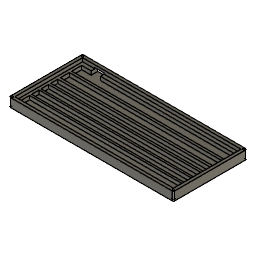
_Bottom_Mech_Case.80a9186b-1b8e-4eee-9d71-97a39b245fca (Autodesk Fusion 360 design; units mm, degrees)
part number: 2026-01-07-15-56-08-248
part number: 2026-01-07-15-57-18-845
Autodesk Fusion 360 part; units mm, degrees
(part 1 of 2)
sketch "Sketch1" plane through (0, 0, 0) normal (0, 0, 1) x (1, 0, 0) in component "MechKeyboard"
  line L0 (0, 0) -> (317.706, 0)
  line L1 (317.706, 0) -> (317.706, 135.488)
  line L2 (317.706, 135.488) -> (0, 135.488)
  line L3 (0, 135.488) -> (0, 0)
  line L4 (-6, -6) -> (323.706, -6)
  line L5 (323.706, -6) -> (323.706, 141.488)
  line L6 (323.706, 141.488) -> (-6, 141.488)
  line L7 (-6, 141.488) -> (-6, -6)
  circle A0 centre (320.206, 137.988) radius 1.7
  circle A1 centre (320.206, 137.988) radius 3
  line L8 (158.853, 135.488) -> (158.853, 141.488) construction
  line L9 (317.706, 67.744) -> (323.706, 67.744) construction
  circle A2 centre (320.206, -2.5) radius 3
  circle A3 centre (320.206, -2.5) radius 1.7
  circle A4 centre (-2.5, 137.988) radius 1.7
  circle A5 centre (-2.5, 137.988) radius 3
  circle A6 centre (-2.5, -2.5) radius 1.7
  circle A7 centre (-2.5, -2.5) radius 3
  dimension "d1" = 317.706
  dimension "d2" = 135.488
  dimension "d3" = 6
  dimension "d4" = 3.4
  dimension "d5" = 3.5
  dimension "d6" = 3.5
  dimension "d7" = 6
  constraint horizontal L0
  constraint vertical L1
  constraint horizontal L2
  constraint vertical L3
  constraint coincident L0.start L3.end
  constraint concentric A0 A1
  constraint midpoint L2 L8.start
  constraint midpoint L6 L8.end
  constraint midpoint L1 L9.start
  constraint midpoint L5 L9.end
  constraint symmetric A0 L9 A3
  constraint symmetric A1 L9 A2
  constraint symmetric A0 L8 A4
  constraint symmetric A1 L8 A5
  constraint symmetric L8 A2 A7
  constraint symmetric L8 A3 A6
  measures "d1" distance of L0.start L0.end
  measures "d2" distance of L0.end L1.end
  measures "d4" diameter of A0
  measures "d5" distance of L5 A0.centre
  measures "d6" distance of L6 A0.centre
  measures "d7" diameter of A1
extrude "Extrude1" add sketch "Sketch1" along normal blind 14.4 from surface at 3.1 contours A1 | A2 | A5 | A7 makes body 1 at (0.4851, -2.7987, 7.9) makes body 2 at (318.8374, 0.1696, 12.7) makes body 3 at (-5.3191, 139.0141, 12.7) makes body 4 at (321.4399, 140.7225, 12.7) in component "MechKeyboard"
extrude "Extrude2" add sketch "Sketch1" along normal blind 17.5 contours L4 L5 L6 L7 bodies 1 2 3 4 in component "MechKeyboard"
extrude "Extrude3" add sketch "Sketch1" along normal blind 3 contours L0 L1 L2 L3 bodies 1 in component "MechKeyboard"
sketch "Sketch1 (2)" plane through (0, 0, 17.5) normal (0, 0, 1) x (-1, 0, 0)
  line L0 (0, 0) -> (0, -135.488)
  line L1 (0, -135.488) -> (-317.706, -135.488)
  line L2 (-317.706, -135.488) -> (-317.706, 0)
  line L3 (-317.706, 0) -> (0, 0)
  line L4 (6, -141.488) -> (6, 6)
  line L5 (6, 6) -> (-323.706, 6)
  line L6 (-323.706, 6) -> (-323.706, -141.488)
  line L7 (-323.706, -141.488) -> (6, -141.488)
  line L8 (-24.5, -141.488) -> (-43, -141.488)
  line L9 (-43, -141.488) -> (-43, -135.488)
  line L10 (-43, -135.488) -> (-24.5, -135.488)
  line L11 (-24.5, -135.488) -> (-24.5, -141.488)
  circle A0 centre (2.5, 2.5) radius 1.7
  circle A1 centre (-320.206, -137.988) radius 1.7
  circle A2 centre (-320.206, 2.5) radius 1.7
  circle A3 centre (2.5, -137.988) radius 1.7
  dimension "d15" = 18.5
  dimension "d17" = 24.5
  constraint horizontal L8
  constraint vertical L9
  constraint horizontal L10
  constraint vertical L11
  constraint coincident L1 L9.end
  constraint coincident L7 L8.start
  measures "d15" distance of L9 L11
  measures "d17" distance of L0.end L11
extrude "Extrude4" cut sketch "Sketch1 (2)" against normal up to surface (9.5 mm away) from surface at -5 contours L1 L7 L8 L9 L10 L11 bodies 1 in component "MechKeyboard"
fillet "Fillet1" radius 2.5 4 edges at (-6, 141.488, 8.75) (-6, -6, 8.75) (323.706, -6, 8.75) (323.706, 141.488, 8.75) on bodies 1 in component "MechKeyboard"
sketch "Sketch2" plane through (0, 0, 3) normal (0, 0, 1) x (-1, 0, 0)
  line L0 (-95.203, -110.7503, 10) -> (-108.203, -110.7503, 10)
  arc A0 through (-232.028, -10.7378, 10) (-232.3816, -10.8842, 10) (-232.528, -11.2378, 10)
  arc A1 through (-184.4218, -23.7378, 10) (-184.0682, -23.5913, 10) (-183.9218, -23.2378, 10)
  arc A2 through (-270.128, -10.7378, 10) (-270.4816, -10.8842, 10) (-270.628, -11.2378, 10)
  arc A3 through (-58.9843, -11.2378, 10) (-59.1307, -10.8842, 10) (-59.4843, -10.7378, 10)
  arc A4 through (-183.9218, -9.2378, 10) (-184.0682, -8.8842, 10) (-184.4218, -8.7378, 10)
  arc A5 through (-308.228, -10.7378, 10) (-308.5816, -10.8842, 10) (-308.728, -11.2378, 10)
  arc A6 through (-251.078, -10.7378, 10) (-251.4316, -10.8842, 10) (-251.578, -11.2378, 10)
  arc A7 through (-11.3593, -11.2378, 10) (-11.5057, -10.8842, 10) (-11.8593, -10.7378, 10)
  arc A8 through (-308.728, -24.2378, 10) (-308.5816, -24.5913, 10) (-308.228, -24.7378, 10)
  arc A9 through (-190.4218, -8.7378, 10) (-190.7753, -8.8842, 10) (-190.9218, -9.2378, 10)
  arc A10 through (-256.628, -11.2378, 10) (-256.7744, -10.8842, 10) (-257.128, -10.7378, 10)
  arc A11 through (-130.4218, -11.2378, 10) (-130.5682, -10.8842, 10) (-130.9218, -10.7378, 10)
  circle A12 through (-323.206, 2.5, 10) (-318.706, -0.0981, 10) (-318.706, 5.0981, 10)
  arc A13 through (-25.3593, -24.2378, 10) (-25.2128, -24.5913, 10) (-24.8593, -24.7378, 10)
  arc A14 through (-275.678, -30.2878, 10) (-275.8244, -29.9342, 10) (-276.178, -29.7878, 10)
  arc A15 through (-289.178, -29.7878, 10) (-289.5316, -29.9342, 10) (-289.678, -30.2878, 10)
  arc A16 through (-295.228, -24.7378, 10) (-294.8744, -24.5913, 10) (-294.728, -24.2378, 10)
  arc A17 through (-294.728, -11.2378, 10) (-294.8744, -10.8842, 10) (-295.228, -10.7378, 10)
  arc A18 through (-295.228, -43.7878, 10) (-294.8744, -43.6413, 10) (-294.728, -43.2878, 10)
  arc A19 through (-289.678, -43.2878, 10) (-289.5316, -43.6413, 10) (-289.178, -43.7878, 10)
  arc A20 through (-185.6905, -43.7878, 10) (-185.3369, -43.6413, 10) (-185.1905, -43.2878, 10)
  arc A21 through (-18.9463, -27.7878, 10) (-19.2998, -27.9342, 10) (-19.4463, -28.2878, 10)
  arc A22 through (-276.178, -43.7878, 10) (-275.8244, -43.6413, 10) (-275.678, -43.2878, 10)
  arc A23 through (-12.9463, -42.7878, 10) (-12.5927, -42.6413, 10) (-12.4463, -42.2878, 10)
  arc A24 through (-249.9843, -43.7878, 10) (-249.6307, -43.6413, 10) (-249.4843, -43.2878, 10)
  arc A25 through (-249.4843, -30.2878, 10) (-249.6307, -29.9342, 10) (-249.9843, -29.7878, 10)
  arc A26 through (-84.3905, -29.7878, 10) (-84.7441, -29.9342, 10) (-84.8905, -30.2878, 10)
  arc A27 through (-83.9218, -9.2378, 10) (-84.0682, -8.8842, 10) (-84.4218, -8.7378, 10)
  arc A28 through (-190.9218, -23.2378, 10) (-190.7753, -23.5913, 10) (-190.4218, -23.7378, 10)
  arc A29 through (-204.2405, -30.2878, 10) (-204.3869, -29.9342, 10) (-204.7405, -29.7878, 10)
  arc A30 through (-143.9218, -10.7378, 10) (-144.2753, -10.8842, 10) (-144.4218, -11.2378, 10)
  arc A31 through (-185.1905, -30.2878, 10) (-185.3369, -29.9342, 10) (-185.6905, -29.7878, 10)
  arc A32 through (-103.9405, -43.2878, 10) (-103.7941, -43.6413, 10) (-103.4405, -43.7878, 10)
  arc A33 through (-48.6718, -10.7378, 10) (-49.0253, -10.8842, 10) (-49.1718, -11.2378, 10)
  arc A34 through (-170.6155, -62.3378, 10) (-170.4691, -62.6913, 10) (-170.1155, -62.8378, 10)
  arc A35 through (-65.3405, -29.7878, 10) (-65.6941, -29.9342, 10) (-65.8405, -30.2878, 10)
  arc A36 through (-279.7098, -61.8378, 10) (-279.3562, -61.6913, 10) (-279.2098, -61.3378, 10)
  arc A37 through (-232.8155, -49.3378, 10) (-232.9619, -48.9842, 10) (-233.3155, -48.8378, 10)
  arc A38 through (-308.728, -62.3378, 10) (-308.5816, -62.6913, 10) (-308.228, -62.8378, 10)
  arc A39 through (-217.7405, -29.7878, 10) (-218.0941, -29.9342, 10) (-218.2405, -30.2878, 10)
  arc A40 through (-118.5155, -49.3378, 10) (-118.6619, -48.9842, 10) (-119.0155, -48.8378, 10)
  arc A41 through (-219.028, -24.7378, 10) (-218.6744, -24.5913, 10) (-218.528, -24.2378, 10)
  arc A42 through (-208.7155, -62.3378, 10) (-208.5691, -62.6913, 10) (-208.2155, -62.8378, 10)
  arc A43 through (-113.4655, -62.3378, 10) (-113.3191, -62.6913, 10) (-112.9655, -62.8378, 10)
  arc A44 through (-198.6905, -29.7878, 10) (-199.0441, -29.9342, 10) (-199.1905, -30.2878, 10)
  arc A45 through (-29.6218, -48.8378, 10) (-29.9753, -48.9842, 10) (-30.1218, -49.3378, 10)
  arc A46 through (-212.978, -10.7378, 10) (-213.3316, -10.8842, 10) (-213.478, -11.2378, 10)
  arc A47 through (-180.1405, -43.2878, 10) (-179.9941, -43.6413, 10) (-179.6405, -43.7878, 10)
  arc A48 through (-80.4155, -49.3378, 10) (-80.5619, -48.9842, 10) (-80.9155, -48.8378, 10)
  arc A49 through (-61.8655, -62.8378, 10) (-61.5119, -62.6913, 10) (-61.3655, -62.3378, 10)
  arc A50 through (-99.9655, -62.8378, 10) (-99.6119, -62.6913, 10) (-99.4655, -62.3378, 10)
  arc A51 through (-208.2155, -48.8378, 10) (-208.5691, -48.9842, 10) (-208.7155, -49.3378, 10)
  arc A52 through (-209.003, -68.3878, 10) (-209.1494, -68.0342, 10) (-209.503, -67.8878, 10)
  arc A53 through (-175.6655, -49.3378, 10) (-175.8119, -48.9842, 10) (-176.1655, -48.8378, 10)
  arc A54 through (-90.4218, -8.7378, 10) (-90.7753, -8.8842, 10) (-90.9218, -9.2378, 10)
  arc A55 through (-199.1905, -43.2878, 10) (-199.0441, -43.6413, 10) (-198.6905, -43.7878, 10)
  arc A56 through (-147.0905, -30.2878, 10) (-147.2369, -29.9342, 10) (-147.5905, -29.7878, 10)
  arc A57 through (-228.053, -68.3878, 10) (-228.1994, -68.0342, 10) (-228.553, -67.8878, 10)
  arc A58 through (-16.6218, -62.8378, 10) (-16.2682, -62.6913, 10) (-16.1218, -62.3378, 10)
  arc A59 through (-72.4843, -10.7378, 10) (-72.8378, -10.8842, 10) (-72.9843, -11.2378, 10)
  arc A60 through (-270.9155, -68.3878, 10) (-271.0619, -68.0342, 10) (-271.4155, -67.8878, 10)
  arc A61 through (-246.3155, -48.8378, 10) (-246.6691, -48.9842, 10) (-246.8155, -49.3378, 10)
  arc A62 through (-223.7905, -43.7878, 10) (-223.4369, -43.6413, 10) (-223.2905, -43.2878, 10)
  arc A63 through (-228.553, -81.8878, 10) (-228.1994, -81.7413, 10) (-228.053, -81.3878, 10)
  arc A64 through (-190.453, -81.8878, 10) (-190.0994, -81.7413, 10) (-189.953, -81.3878, 10)
  arc A65 through (-95.203, -81.8878, 10) (-94.8494, -81.7413, 10) (-94.703, -81.3878, 10)
  arc A66 through (-166.6405, -43.7878, 10) (-166.2869, -43.6413, 10) (-166.1405, -43.2878, 10)
  arc A67 through (-165.353, -67.8878, 10) (-165.7066, -68.0342, 10) (-165.853, -68.3878, 10)
  arc A68 through (-170.1155, -48.8378, 10) (-170.4691, -48.9842, 10) (-170.6155, -49.3378, 10)
  arc A69 through (-90.4405, -43.7878, 10) (-90.0869, -43.6413, 10) (-89.9405, -43.2878, 10)
  arc A70 through (-89.153, -67.8878, 10) (-89.5066, -68.0342, 10) (-89.653, -68.3878, 10)
  arc A71 through (-146.303, -67.8878, 10) (-146.6566, -68.0342, 10) (-146.803, -68.3878, 10)
  arc A72 through (-38.053, -81.8878, 10) (-37.6994, -81.7413, 10) (-37.553, -81.3878, 10)
  arc A73 through (-70.103, -67.8878, 10) (-70.4566, -68.0342, 10) (-70.603, -68.3878, 10)
  arc A74 through (-146.803, -81.3878, 10) (-146.6566, -81.7413, 10) (-146.303, -81.8878, 10)
  arc A75 through (-132.0155, -48.8378, 10) (-132.3691, -48.9842, 10) (-132.5155, -49.3378, 10)
  line L1 (-58.9843, -24.2378, 10) -> (-58.9843, -11.2378, 10)
  line L2 (-72.9843, -24.2378, 10) -> (-72.9843, -11.2378, 10)
  arc A76 through (-70.603, -81.3878, 10) (-70.4566, -81.7413, 10) (-70.103, -81.8878, 10)
  arc A77 through (-95.203, -124.7503, 10) (-94.8494, -124.6038, 10) (-94.703, -124.2503, 10)
  arc A78 through (-89.653, -124.2503, 10) (-89.5066, -124.6038, 10) (-89.153, -124.7503, 10)
  line L3 (-190.9218, -23.2378, 10) -> (-190.9218, -9.2378, 10)
  arc A79 through (-165.853, -81.3878, 10) (-165.7066, -81.7413, 10) (-165.353, -81.8878, 10)
  line L4 (-59.4843, -24.7378, 10) -> (-72.4843, -24.7378, 10)
  arc A80 through (-209.503, -81.8878, 10) (-209.1494, -81.7413, 10) (-209.003, -81.3878, 10)
  arc A81 through (-57.103, -124.7503, 10) (-56.7494, -124.6038, 10) (-56.603, -124.2503, 10)
  arc A82 through (-127.753, -81.3878, 10) (-127.6066, -81.7413, 10) (-127.253, -81.8878, 10)
  line L5 (-84.4218, -8.7378, 10) -> (-90.4218, -8.7378, 10)
  line L6 (-35.6718, -24.7378, 10) -> (-48.6718, -24.7378, 10)
  line L7 (-256.628, -24.2378, 10) -> (-256.628, -11.2378, 10)
  arc A83 through (-264.215, -84.9378, 10) (-264.5686, -85.0842, 10) (-264.715, -85.4378, 10)
  line L8 (-323.706, 6, 10) -> (-323.706, -141.488, 10)
  arc A84 through (-232.528, -100.4378, 10) (-232.3816, -100.7913, 10) (-232.028, -100.9378, 10)
  arc A85 through (-266.153, -87.4378, 10) (-266.2994, -87.0842, 10) (-266.653, -86.9378, 10)
  line L9 (-289.678, -43.2878, 10) -> (-289.678, -30.2878, 10)
  line L10 (-275.678, -43.2878, 10) -> (-275.678, -30.2878, 10)
  line L11 (-289.678, -24.2378, 10) -> (-289.678, -11.2378, 10)
  line L12 (-90.9218, -23.2378, 10) -> (-90.9218, -9.2378, 10)
  line L13 (-59.4843, -10.7378, 10) -> (-72.4843, -10.7378, 10)
  arc A86 through (-123.278, -87.4378, 10) (-123.4244, -87.0842, 10) (-123.778, -86.9378, 10)
  line L14 (-183.9218, -23.2378, 10) -> (-183.9218, -9.2378, 10)
  line L15 (-223.2905, -43.2878, 10) -> (-223.2905, -30.2878, 10)
  line L16 (-180.1405, -43.2878, 10) -> (-180.1405, -30.2878, 10)
  line L17 (-204.2405, -43.2878, 10) -> (-204.2405, -30.2878, 10)
  line L18 (-218.2405, -43.2878, 10) -> (-218.2405, -30.2878, 10)
  line L19 (-308.728, -43.2878, 10) -> (-308.728, -30.2878, 10)
  arc A87 through (-161.378, -87.4378, 10) (-161.5244, -87.0842, 10) (-161.878, -86.9378, 10)
  arc A88 through (-47.078, -87.4378, 10) (-47.2244, -87.0842, 10) (-47.578, -86.9378, 10)
  line L20 (-130.4218, -24.2378, 10) -> (-130.4218, -11.2378, 10)
  line L21 (-84.8905, -43.2878, 10) -> (-84.8905, -30.2878, 10)
  line L22 (-36.8223, -42.7878, 10) -> (-42.8223, -42.7878, 10)
  arc A89 through (-8.978, -87.4378, 10) (-9.1244, -87.0842, 10) (-9.478, -86.9378, 10)
  arc A90 through (-22.978, -100.4378, 10) (-22.8316, -100.7913, 10) (-22.478, -100.9378, 10)
  line L23 (-161.0905, -43.2878, 10) -> (-161.0905, -30.2878, 10)
  line L24 (-109.4905, -29.7878, 10) -> (-122.4905, -29.7878, 10)
  line L25 (-128.0405, -43.2878, 10) -> (-128.0405, -30.2878, 10)
  line L26 (-147.5905, -29.7878, 10) -> (-160.5905, -29.7878, 10)
  line L27 (-42.8155, -62.8378, 10) -> (-55.8155, -62.8378, 10)
  line L28 (-70.603, -81.3878, 10) -> (-70.603, -68.3878, 10)
  line L29 (-38.053, -81.8878, 10) -> (-51.053, -81.8878, 10)
  line L30 (-16.1218, -62.3378, 10) -> (-16.1218, -49.3378, 10)
  line L31 (-119.0155, -48.8378, 10) -> (-132.0155, -48.8378, 10)
  line L32 (-11.3593, -24.2378, 10) -> (-11.3593, -11.2378, 10)
  line L33 (-308.728, -81.3878, 10) -> (-308.728, -68.3878, 10)
  line L34 (-157.1155, -48.8378, 10) -> (-170.1155, -48.8378, 10)
  line L35 (-42.3155, -62.3378, 10) -> (-42.3155, -49.3378, 10)
  line L36 (-51.553, -81.3878, 10) -> (-51.553, -68.3878, 10)
  line L37 (-249.9843, -43.7878, 10) -> (-262.9843, -43.7878, 10)
  line L38 (-80.9155, -62.8378, 10) -> (-93.9155, -62.8378, 10)
  line L39 (-109.4905, -43.7878, 10) -> (-122.4905, -43.7878, 10)
  line L40 (-288.591, -99.4378, 10) -> (-288.591, -85.4378, 10)
  line L41 (-30.1218, -62.3378, 10) -> (-30.1218, -49.3378, 10)
  line L42 (-133.303, -81.8878, 10) -> (-146.303, -81.8878, 10)
  line L43 (-266.653, -100.9378, 10) -> (-279.653, -100.9378, 10)
  line L44 (-228.053, -81.3878, 10) -> (-228.053, -68.3878, 10)
  line L45 (-165.853, -81.3878, 10) -> (-165.853, -68.3878, 10)
  line L46 (-12.9463, -42.7878, 10) -> (-18.9463, -42.7878, 10)
  line L47 (-52.3405, -29.7878, 10) -> (-65.3405, -29.7878, 10)
  line L48 (-270.9155, -81.3878, 10) -> (-270.9155, -68.3878, 10)
  line L49 (-76.153, -67.8878, 10) -> (-89.153, -67.8878, 10)
  line L50 (-295.228, -81.8878, 10) -> (-308.228, -81.8878, 10)
  line L51 (-118.228, -100.4378, 10) -> (-118.228, -87.4378, 10)
  line L52 (-295.228, -67.8878, 10) -> (-308.228, -67.8878, 10)
  line L53 (-199.978, -100.9378, 10) -> (-212.978, -100.9378, 10)
  line L54 (-295.228, -86.9378, 10) -> (-308.228, -86.9378, 10)
  line L55 (-99.178, -100.4378, 10) -> (-99.178, -87.4378, 10)
  line L56 (-108.703, -81.3878, 10) -> (-108.703, -68.3878, 10)
  line L57 (-20.8843, -43.2878, 10) -> (-20.8843, -30.2878, 10)
  line L58 (-199.478, -100.4378, 10) -> (-199.478, -87.4378, 10)
  arc A91 through (-289.678, -24.2378, 10) (-289.5316, -24.5913, 10) (-289.178, -24.7378, 10)
  circle A92 through (-0.5, -137.988, 10) (4, -140.5861, 10) (4, -135.3899, 10)
  arc A93 through (-251.078, -86.9378, 10) (-251.4316, -87.0842, 10) (-251.578, -87.4378, 10)
  line L59 (-108.703, -124.2503, 10) -> (-108.703, -111.2503, 10)
  arc A94 through (-281.591, -85.4378, 10) (-281.7374, -85.0842, 10) (-282.091, -84.9378, 10)
  arc A95 through (-257.715, -85.4378, 10) (-257.8614, -85.0842, 10) (-258.215, -84.9378, 10)
  arc A96 through (-42.8155, -62.8378, 10) (-42.4619, -62.6913, 10) (-42.3155, -62.3378, 10)
  arc A97 through (-70.8905, -30.2878, 10) (-71.0369, -29.9342, 10) (-71.3905, -29.7878, 10)
  arc A98 through (-114.253, -81.8878, 10) (-113.8994, -81.7413, 10) (-113.753, -81.3878, 10)
  arc A99 through (-19.4463, -42.2878, 10) (-19.2998, -42.6413, 10) (-18.9463, -42.7878, 10)
  arc A100 through (-65.8405, -43.2878, 10) (-65.6941, -43.6413, 10) (-65.3405, -43.7878, 10)
  arc A101 through (-13.7405, -68.3878, 10) (-13.8869, -68.0342, 10) (-14.2405, -67.8878, 10)
  arc A102 through (-308.228, -67.8878, 10) (-308.5816, -68.0342, 10) (-308.728, -68.3878, 10)
  arc A103 through (-219.028, -100.9378, 10) (-218.6744, -100.7913, 10) (-218.528, -100.4378, 10)
  arc A104 through (-27.7405, -81.3878, 10) (-27.5941, -81.7413, 10) (-27.2405, -81.8878, 10)
  arc A105 through (-295.228, -81.8878, 10) (-294.8744, -81.7413, 10) (-294.728, -81.3878, 10)
  arc A106 through (-34.8843, -43.2878, 10) (-34.7378, -43.6413, 10) (-34.3843, -43.7878, 10)
  arc A107 through (-142.828, -100.9378, 10) (-142.4744, -100.7913, 10) (-142.328, -100.4378, 10)
  arc A108 through (-56.603, -68.3878, 10) (-56.7494, -68.0342, 10) (-57.103, -67.8878, 10)
  arc A109 through (-117.728, -86.9378, 10) (-118.0816, -87.0842, 10) (-118.228, -87.4378, 10)
  arc A110 through (-9.478, -100.9378, 10) (-9.1244, -100.7913, 10) (-8.978, -100.4378, 10)
  arc A111 through (-257.128, -124.7503, 10) (-256.7744, -124.6038, 10) (-256.628, -124.2503, 10)
  arc A112 through (-238.078, -100.9378, 10) (-237.7244, -100.7913, 10) (-237.578, -100.4378, 10)
  arc A113 through (-282.091, -99.9378, 10) (-281.7374, -99.7913, 10) (-281.591, -99.4378, 10)
  line L60 (-9.478, -110.7503, 10) -> (-22.478, -110.7503, 10)
  arc A114 through (-251.578, -100.4378, 10) (-251.4316, -100.7913, 10) (-251.078, -100.9378, 10)
  arc A115 through (-79.628, -86.9378, 10) (-79.9816, -87.0842, 10) (-80.128, -87.4378, 10)
  arc A116 through (-246.8155, -62.3378, 10) (-246.6691, -62.6913, 10) (-246.3155, -62.8378, 10)
  arc A117 through (-157.1155, -62.8378, 10) (-156.7619, -62.6913, 10) (-156.6155, -62.3378, 10)
  arc A118 through (-80.9155, -62.8378, 10) (-80.5619, -62.6913, 10) (-80.4155, -62.3378, 10)
  arc A119 through (-285.7098, -46.8378, 10) (-286.0633, -46.9842, 10) (-286.2098, -47.3378, 10)
  arc A120 through (-261.103, -81.3878, 10) (-260.9566, -81.7413, 10) (-260.603, -81.8878, 10)
  arc A121 through (-264.715, -99.4378, 10) (-264.5686, -99.7913, 10) (-264.215, -99.9378, 10)
  arc A122 through (-41.528, -86.9378, 10) (-41.8816, -87.0842, 10) (-42.028, -87.4378, 10)
  arc A123 through (-258.215, -99.9378, 10) (-257.8614, -99.7913, 10) (-257.715, -99.4378, 10)
  arc A124 through (-42.028, -100.4378, 10) (-41.8816, -100.7913, 10) (-41.528, -100.9378, 10)
  arc A125 through (-176.1655, -62.8378, 10) (-175.8119, -62.6913, 10) (-175.6655, -62.3378, 10)
  arc A126 through (-22.478, -86.9378, 10) (-22.8316, -87.0842, 10) (-22.978, -87.4378, 10)
  arc A127 through (-89.653, -81.3878, 10) (-89.5066, -81.7413, 10) (-89.153, -81.8878, 10)
  arc A128 through (-193.928, -86.9378, 10) (-194.2816, -87.0842, 10) (-194.428, -87.4378, 10)
  arc A129 through (-70.603, -124.2503, 10) (-70.4566, -124.6038, 10) (-70.103, -124.7503, 10)
  arc A130 through (-251.578, -124.2503, 10) (-251.4316, -124.6038, 10) (-251.078, -124.7503, 10)
  arc A131 through (-104.728, -100.9378, 10) (-104.3744, -100.7913, 10) (-104.228, -100.4378, 10)
  arc A132 through (-194.7155, -111.2503, 10) (-194.8619, -110.8967, 10) (-195.2155, -110.7503, 10)
  arc A133 through (-247.603, -81.8878, 10) (-247.2494, -81.7413, 10) (-247.103, -81.3878, 10)
  line L61 (-251.578, -24.2378, 10) -> (-251.578, -11.2378, 10)
  arc A134 through (-237.578, -87.4378, 10) (-237.7244, -87.0842, 10) (-238.078, -86.9378, 10)
  arc A135 through (-199.478, -87.4378, 10) (-199.6244, -87.0842, 10) (-199.978, -86.9378, 10)
  arc A136 through (-56.603, -111.2503, 10) (-56.7494, -110.8967, 10) (-57.103, -110.7503, 10)
  arc A137 through (-104.228, -87.4378, 10) (-104.3744, -87.0842, 10) (-104.728, -86.9378, 10)
  arc A138 through (-308.728, -100.4378, 10) (-308.5816, -100.7913, 10) (-308.228, -100.9378, 10)
  arc A139 through (-42.3155, -49.3378, 10) (-42.4619, -48.9842, 10) (-42.8155, -48.8378, 10)
  arc A140 through (-80.128, -100.4378, 10) (-79.9816, -100.7913, 10) (-79.628, -100.9378, 10)
  arc A141 through (-151.5655, -124.2503, 10) (-151.4191, -124.6038, 10) (-151.0655, -124.7503, 10)
  arc A142 through (-75.3655, -62.3378, 10) (-75.2191, -62.6913, 10) (-74.8655, -62.8378, 10)
  arc A143 through (-57.103, -81.8878, 10) (-56.7494, -81.7413, 10) (-56.603, -81.3878, 10)
  arc A144 through (-175.6655, -111.2503, 10) (-175.8119, -110.8967, 10) (-176.1655, -110.7503, 10)
  arc A145 through (-76.153, -81.8878, 10) (-75.7994, -81.7413, 10) (-75.653, -81.3878, 10)
  arc A146 through (-75.653, -111.2503, 10) (-75.7994, -110.8967, 10) (-76.153, -110.7503, 10)
  arc A147 through (-276.178, -124.7503, 10) (-275.8244, -124.6038, 10) (-275.678, -124.2503, 10)
  line L62 (-323.706, -141.488, 10) -> (6, -141.488, 10)
  arc A148 through (-308.728, -81.3878, 10) (-308.5816, -81.7413, 10) (-308.228, -81.8878, 10)
  arc A149 through (-60.578, -86.9378, 10) (-60.9316, -87.0842, 10) (-61.078, -87.4378, 10)
  arc A150 through (-242.053, -81.3878, 10) (-241.9066, -81.7413, 10) (-241.553, -81.8878, 10)
  arc A151 through (-157.1155, -124.7503, 10) (-156.7619, -124.6038, 10) (-156.6155, -124.2503, 10)
  arc A152 through (-208.2155, -110.7503, 10) (-208.5691, -110.8967, 10) (-208.7155, -111.2503, 10)
  line L63 (-238.078, -24.7378, 10) -> (-251.078, -24.7378, 10)
  line L64 (-238.078, -10.7378, 10) -> (-251.078, -10.7378, 10)
  line L65 (-218.528, -24.2378, 10) -> (-218.528, -11.2378, 10)
  arc A153 through (-137.5655, -111.2503, 10) (-137.7119, -110.8967, 10) (-138.0655, -110.7503, 10)
  arc A154 through (-222.503, -67.8878, 10) (-222.8566, -68.0342, 10) (-223.003, -68.3878, 10)
  arc A155 through (-108.203, -110.7503, 10) (-108.5566, -110.8967, 10) (-108.703, -111.2503, 10)
  line L66 (-294.728, -62.3378, 10) -> (-294.728, -49.3378, 10)
  line L67 (-255.8338, -46.8378, 10) -> (-261.8338, -46.8378, 10)
  line L68 (-277.7718, -62.3378, 10) -> (-277.7718, -49.3378, 10)
  line L69 (-18.3593, -10.7378, 10) -> (-18.3593, 6, 10) construction
  line L70 (-70.8905, -43.2878, 10) -> (-70.8905, -30.2878, 10)
  arc A156 through (-127.753, -124.2503, 10) (-127.6066, -124.6038, 10) (-127.253, -124.7503, 10)
  line L71 (-71.3905, -43.7878, 10) -> (-84.3905, -43.7878, 10)
  line L72 (-36.8223, -27.7878, 10) -> (-42.8223, -27.7878, 10)
  line L73 (-80.4155, -62.3378, 10) -> (-80.4155, -49.3378, 10)
  arc A157 through (-70.103, -110.7503, 10) (-70.4566, -110.8967, 10) (-70.603, -111.2503, 10)
  line L74 (-36.3223, -42.2878, 10) -> (-36.3223, -28.2878, 10)
  line L75 (-176.1655, -62.8378, 10) -> (-189.1655, -62.8378, 10)
  line L76 (-233.3155, -48.8378, 10) -> (-246.3155, -48.8378, 10)
  line L77 (-276.178, -24.7378, 10) -> (-289.178, -24.7378, 10)
  line L78 (-264.2718, -62.8378, 10) -> (-277.2718, -62.8378, 10)
  line L79 (-151.5655, -62.3378, 10) -> (-151.5655, -49.3378, 10)
  line L80 (-94.4155, -62.3378, 10) -> (-94.4155, -49.3378, 10)
  line L81 (-264.2718, -48.8378, 10) -> (-277.2718, -48.8378, 10)
  line L82 (-294.728, -24.2378, 10) -> (-294.728, -11.2378, 10)
  line L83 (-262.3338, -61.3378, 10) -> (-262.3338, -47.3378, 10)
  line L84 (-246.8155, -62.3378, 10) -> (-246.8155, -49.3378, 10)
  line L85 (-228.553, -81.8878, 10) -> (-241.553, -81.8878, 10)
  line L86 (-257.128, -10.7378, 10) -> (-270.128, -10.7378, 10)
  line L87 (-184.4218, -23.7378, 10) -> (-190.4218, -23.7378, 10)
  line L88 (-90.4405, -43.7878, 10) -> (-103.4405, -43.7878, 10)
  line L89 (-194.7155, -62.3378, 10) -> (-194.7155, -49.3378, 10)
  line L90 (-90.4405, -29.7878, 10) -> (-103.4405, -29.7878, 10)
  arc A158 through (-270.128, -110.7503, 10) (-270.4816, -110.8967, 10) (-270.628, -111.2503, 10)
  arc A159 through (-238.078, -124.7503, 10) (-237.7244, -124.6038, 10) (-237.578, -124.2503, 10)
  line L91 (-185.1905, -43.2878, 10) -> (-185.1905, -30.2878, 10)
  arc A160 through (-232.528, -124.2503, 10) (-232.3816, -124.6038, 10) (-232.028, -124.7503, 10)
  arc A161 through (-138.0655, -124.7503, 10) (-137.7119, -124.6038, 10) (-137.5655, -124.2503, 10)
  arc A162 through (-113.753, -111.2503, 10) (-113.8994, -110.8967, 10) (-114.253, -110.7503, 10)
  line L92 (-108.9905, -43.2878, 10) -> (-108.9905, -30.2878, 10)
  circle A163 through (-323.206, -137.988, 10) (-318.706, -140.5861, 10) (-318.706, -135.3899, 10)
  arc A164 through (-238.078, -24.7378, 10) (-237.7244, -24.5913, 10) (-237.578, -24.2378, 10)
  arc A165 through (-218.528, -11.2378, 10) (-218.6744, -10.8842, 10) (-219.028, -10.7378, 10)
  arc A166 through (-199.478, -11.2378, 10) (-199.6244, -10.8842, 10) (-199.978, -10.7378, 10)
  arc A167 through (-130.9218, -24.7378, 10) (-130.5682, -24.5913, 10) (-130.4218, -24.2378, 10)
  line L93 (-95.203, -124.7503, 10) -> (-108.203, -124.7503, 10)
  arc A168 through (-90.9218, -23.2378, 10) (-90.7753, -23.5913, 10) (-90.4218, -23.7378, 10)
  line L94 (-127.753, -124.2503, 10) -> (-127.753, -111.2503, 10)
  arc A169 through (-59.4843, -24.7378, 10) (-59.1307, -24.5913, 10) (-58.9843, -24.2378, 10)
  arc A170 through (-237.2905, -43.2878, 10) (-237.1441, -43.6413, 10) (-236.7905, -43.7878, 10)
  line L95 (-22.978, -124.2503, 10) -> (-22.978, -111.2503, 10)
  arc A171 through (-262.9843, -29.7878, 10) (-263.3378, -29.9342, 10) (-263.4843, -30.2878, 10)
  line L96 (-176.1655, -110.7503, 10) -> (-189.1655, -110.7503, 10)
  line L97 (-113.753, -124.2503, 10) -> (-113.753, -111.2503, 10)
  arc A172 through (-141.5405, -29.7878, 10) (-141.8941, -29.9342, 10) (-142.0405, -30.2878, 10)
  line L98 (-308.728, -100.4378, 10) -> (-308.728, -87.4378, 10)
  line L99 (-9.478, -124.7503, 10) -> (-22.478, -124.7503, 10)
  line L100 (-61.078, -100.4378, 10) -> (-61.078, -87.4378, 10)
  line L101 (-9.478, -100.9378, 10) -> (-22.478, -100.9378, 10)
  line L102 (-237.578, -124.2503, 10) -> (-237.578, -111.2503, 10)
  line L103 (-76.153, -124.7503, 10) -> (-89.153, -124.7503, 10)
  line L104 (-89.653, -124.2503, 10) -> (-89.653, -111.2503, 10)
  line L105 (-256.628, -124.2503, 10) -> (-256.628, -111.2503, 10)
  line L106 (-14.2405, -81.8878, 10) -> (-27.2405, -81.8878, 10)
  line L107 (-266.153, -100.4378, 10) -> (-266.153, -87.4378, 10)
  line L108 (-208.7155, -62.3378, 10) -> (-208.7155, -49.3378, 10)
  line L109 (-282.091, -84.9378, 10) -> (-288.091, -84.9378, 10)
  line L110 (-175.6655, -62.3378, 10) -> (-175.6655, -49.3378, 10)
  line L111 (-238.078, -110.7503, 10) -> (-251.078, -110.7503, 10)
  line L112 (-258.215, -84.9378, 10) -> (-264.215, -84.9378, 10)
  line L113 (-218.528, -100.4378, 10) -> (-218.528, -87.4378, 10)
  line L114 (-161.378, -100.4378, 10) -> (-161.378, -87.4378, 10)
  line L115 (-104.228, -100.4378, 10) -> (-104.228, -87.4378, 10)
  line L116 (-66.628, -100.9378, 10) -> (-79.628, -100.9378, 10)
  line L117 (-161.878, -100.9378, 10) -> (-174.878, -100.9378, 10)
  line L118 (-180.928, -86.9378, 10) -> (-193.928, -86.9378, 10)
  line L119 (-175.378, -100.4378, 10) -> (-175.378, -87.4378, 10)
  line L120 (-104.728, -100.9378, 10) -> (-117.728, -100.9378, 10)
  line L121 (-16.6218, -48.8378, 10) -> (-29.6218, -48.8378, 10)
  line L122 (-42.028, -100.4378, 10) -> (-42.028, -87.4378, 10)
  line L123 (-289.678, -124.2503, 10) -> (-289.678, -111.2503, 10)
  line L124 (-42.8155, -48.8378, 10) -> (-55.8155, -48.8378, 10)
  line L125 (-80.9155, -48.8378, 10) -> (-93.9155, -48.8378, 10)
  line L126 (-85.178, -100.4378, 10) -> (-85.178, -87.4378, 10)
  line L127 (-57.103, -110.7503, 10) -> (-70.103, -110.7503, 10)
  line L128 (-146.803, -81.3878, 10) -> (-146.803, -68.3878, 10)
  line L129 (-238.078, -124.7503, 10) -> (-251.078, -124.7503, 10)
  line L130 (-247.603, -81.8878, 10) -> (-260.603, -81.8878, 10)
  line L131 (-170.6155, -124.2503, 10) -> (-170.6155, -111.2503, 10)
  line L132 (-156.6155, -124.2503, 10) -> (-156.6155, -111.2503, 10)
  line L133 (-95.203, -81.8878, 10) -> (-108.203, -81.8878, 10)
  line L134 (-75.653, -124.2503, 10) -> (-75.653, -111.2503, 10)
  line L135 (-95.203, -67.8878, 10) -> (-108.203, -67.8878, 10)
  line L136 (-214.2655, -48.8378, 10) -> (-227.2655, -48.8378, 10)
  line L137 (-214.2655, -62.8378, 10) -> (-227.2655, -62.8378, 10)
  line L138 (-295.228, -48.8378, 10) -> (-308.228, -48.8378, 10)
  line L139 (-190.453, -81.8878, 10) -> (-203.453, -81.8878, 10)
  line L140 (-194.428, -100.4378, 10) -> (-194.428, -87.4378, 10)
  line L141 (-37.553, -81.3878, 10) -> (-37.553, -68.3878, 10)
  line L142 (-28.528, -100.9378, 10) -> (-41.528, -100.9378, 10)
  line L143 (-113.753, -81.3878, 10) -> (-113.753, -68.3878, 10)
  line L144 (-8.978, -100.4378, 10) -> (-8.978, -87.4378, 10)
  line L145 (-157.1155, -62.8378, 10) -> (-170.1155, -62.8378, 10)
  arc A173 through (-194.7155, -49.3378, 10) (-194.8619, -48.9842, 10) (-195.2155, -48.8378, 10)
  arc A174 through (-12.4463, -28.2878, 10) (-12.5927, -27.9342, 10) (-12.9463, -27.7878, 10)
  arc A175 through (-98.678, -86.9378, 10) (-99.0316, -87.0842, 10) (-99.178, -87.4378, 10)
  line L146 (-249.9843, -29.7878, 10) -> (-262.9843, -29.7878, 10)
  line L147 (-21.3843, -29.7878, 10) -> (-34.3843, -29.7878, 10)
  line L148 (-261.103, -81.3878, 10) -> (-261.103, -68.3878, 10)
  arc A176 through (-99.178, -100.4378, 10) (-99.0316, -100.7913, 10) (-98.678, -100.9378, 10)
  arc A177 through (-93.9155, -48.8378, 10) (-94.2691, -48.9842, 10) (-94.4155, -49.3378, 10)
  line L149 (-170.6155, -62.3378, 10) -> (-170.6155, -49.3378, 10)
  arc A178 through (-255.8338, -61.8378, 10) (-255.4802, -61.6913, 10) (-255.3338, -61.3378, 10)
  line L150 (-228.553, -67.8878, 10) -> (-241.553, -67.8878, 10)
  arc A179 through (-28.528, -100.9378, 10) (-28.1744, -100.7913, 10) (-28.028, -100.4378, 10)
  arc A180 through (-264.2718, -62.8378, 10) (-263.9182, -62.6913, 10) (-263.7718, -62.3378, 10)
  arc A181 through (-30.1218, -62.3378, 10) (-29.9753, -62.6913, 10) (-29.6218, -62.8378, 10)
  line L151 (-56.603, -81.3878, 10) -> (-56.603, -68.3878, 10)
  arc A182 through (-295.228, -62.8378, 10) (-294.8744, -62.6913, 10) (-294.728, -62.3378, 10)
  line L152 (-242.053, -81.3878, 10) -> (-242.053, -68.3878, 10)
  line L153 (-51.8405, -43.2878, 10) -> (-51.8405, -30.2878, 10)
  line L154 (-255.8338, -61.8378, 10) -> (-261.8338, -61.8378, 10)
  arc A183 through (-132.5155, -62.3378, 10) (-132.3691, -62.6913, 10) (-132.0155, -62.8378, 10)
  arc A184 through (-170.6155, -124.2503, 10) (-170.4691, -124.6038, 10) (-170.1155, -124.7503, 10)
  arc A185 through (-284.4155, -67.8878, 10) (-284.7691, -68.0342, 10) (-284.9155, -68.3878, 10)
  line L155 (-61.3655, -62.3378, 10) -> (-61.3655, -49.3378, 10)
  line L156 (-195.2155, -48.8378, 10) -> (-208.2155, -48.8378, 10)
  arc A186 through (-112.9655, -48.8378, 10) (-113.3191, -48.9842, 10) (-113.4655, -49.3378, 10)
  arc A187 through (-213.7655, -49.3378, 10) (-213.9119, -48.9842, 10) (-214.2655, -48.8378, 10)
  line L157 (-99.9655, -62.8378, 10) -> (-112.9655, -62.8378, 10)
  arc A188 through (-214.2655, -62.8378, 10) (-213.9119, -62.6913, 10) (-213.7655, -62.3378, 10)
  line L158 (-213.7655, -62.3378, 10) -> (-213.7655, -49.3378, 10)
  line L159 (-71.3905, -29.7878, 10) -> (-84.3905, -29.7878, 10)
  arc A189 through (-256.628, -111.2503, 10) (-256.7744, -110.8967, 10) (-257.128, -110.7503, 10)
  arc A190 through (-56.3155, -62.3378, 10) (-56.1691, -62.6913, 10) (-55.8155, -62.8378, 10)
  line L160 (-56.3155, -62.3378, 10) -> (-56.3155, -49.3378, 10)
  arc A191 through (-284.9155, -81.3878, 10) (-284.7691, -81.7413, 10) (-284.4155, -81.8878, 10)
  arc A192 through (-170.903, -68.3878, 10) (-171.0494, -68.0342, 10) (-171.403, -67.8878, 10)
  line L161 (-279.7098, -61.8378, 10) -> (-285.7098, -61.8378, 10)
  arc A193 through (-271.4155, -81.8878, 10) (-271.0619, -81.7413, 10) (-270.9155, -81.3878, 10)
  line L162 (-99.9655, -48.8378, 10) -> (-112.9655, -48.8378, 10)
  line L163 (-190.453, -67.8878, 10) -> (-203.453, -67.8878, 10)
  arc A194 through (-89.153, -110.7503, 10) (-89.5066, -110.8967, 10) (-89.653, -111.2503, 10)
  arc A195 through (-127.253, -67.8878, 10) (-127.6066, -68.0342, 10) (-127.753, -68.3878, 10)
  arc A196 through (-295.228, -100.9378, 10) (-294.8744, -100.7913, 10) (-294.728, -100.4378, 10)
  arc A197 through (-132.803, -68.3878, 10) (-132.9494, -68.0342, 10) (-133.303, -67.8878, 10)
  arc A198 through (-133.303, -81.8878, 10) (-132.9494, -81.7413, 10) (-132.803, -81.3878, 10)
  line L164 (-184.903, -81.3878, 10) -> (-184.903, -68.3878, 10)
  arc A199 through (-203.453, -67.8878, 10) (-203.8066, -68.0342, 10) (-203.953, -68.3878, 10)
  line L165 (-189.6655, -62.3378, 10) -> (-189.6655, -49.3378, 10)
  line L166 (-99.4655, -62.3378, 10) -> (-99.4655, -49.3378, 10)
  arc A200 through (-171.403, -81.8878, 10) (-171.0494, -81.7413, 10) (-170.903, -81.3878, 10)
  line L167 (-171.403, -67.8878, 10) -> (-184.403, -67.8878, 10)
  arc A201 through (-212.978, -86.9378, 10) (-213.3316, -87.0842, 10) (-213.478, -87.4378, 10)
  arc A202 through (-16.1218, -49.3378, 10) (-16.2682, -48.9842, 10) (-16.6218, -48.8378, 10)
  line L168 (-128.5405, -43.7878, 10) -> (-141.5405, -43.7878, 10)
  line L169 (-286.2098, -61.3378, 10) -> (-286.2098, -47.3378, 10)
  arc A203 through (-175.378, -100.4378, 10) (-175.2316, -100.7913, 10) (-174.878, -100.9378, 10)
  arc A204 through (-294.728, -87.4378, 10) (-294.8744, -87.0842, 10) (-295.228, -86.9378, 10)
  line L170 (-43.3223, -42.2878, 10) -> (-43.3223, -28.2878, 10)
  arc A205 through (-247.103, -68.3878, 10) (-247.2494, -68.0342, 10) (-247.603, -67.8878, 10)
  arc A206 through (-213.478, -100.4378, 10) (-213.3316, -100.7913, 10) (-212.978, -100.9378, 10)
  arc A207 through (-94.703, -68.3878, 10) (-94.8494, -68.0342, 10) (-95.203, -67.8878, 10)
  line L171 (-263.4843, -43.2878, 10) -> (-263.4843, -30.2878, 10)
  line L172 (-295.228, -62.8378, 10) -> (-308.228, -62.8378, 10)
  line L173 (-35.6718, -10.7378, 10) -> (-48.6718, -10.7378, 10)
  line L174 (-276.178, -43.7878, 10) -> (-289.178, -43.7878, 10)
  line L175 (-308.728, -62.3378, 10) -> (-308.728, -49.3378, 10)
  line L176 (-275.678, -24.2378, 10) -> (-275.678, -11.2378, 10)
  arc A208 through (-94.703, -111.2503, 10) (-94.8494, -110.8967, 10) (-95.203, -110.7503, 10)
  line L177 (-295.228, -29.7878, 10) -> (-308.228, -29.7878, 10)
  arc A209 through (-108.703, -81.3878, 10) (-108.5566, -81.7413, 10) (-108.203, -81.8878, 10)
  line L178 (-52.3405, -43.7878, 10) -> (-65.3405, -43.7878, 10)
  line L179 (6, 6, 10) -> (-323.706, 6, 10)
  line L180 (-128.5405, -29.7878, 10) -> (-141.5405, -29.7878, 10)
  line L181 (-295.228, -10.7378, 10) -> (-308.228, -10.7378, 10)
  line L182 (-199.478, -24.2378, 10) -> (-199.478, -11.2378, 10)
  line L183 (-223.7905, -29.7878, 10) -> (-236.7905, -29.7878, 10)
  line L184 (-199.978, -24.7378, 10) -> (-212.978, -24.7378, 10)
  line L185 (-89.9405, -43.2878, 10) -> (-89.9405, -30.2878, 10)
  line L186 (-279.2098, -61.3378, 10) -> (-279.2098, -47.3378, 10)
  line L187 (-257.128, -24.7378, 10) -> (-270.128, -24.7378, 10)
  line L188 (-227.7655, -62.3378, 10) -> (-227.7655, -49.3378, 10)
  arc A210 through (-174.878, -86.9378, 10) (-175.2316, -87.0842, 10) (-175.378, -87.4378, 10)
  line L189 (-276.178, -29.7878, 10) -> (-289.178, -29.7878, 10)
  line L190 (-147.5905, -43.7878, 10) -> (-160.5905, -43.7878, 10)
  line L191 (-308.728, -93.9378, 10) -> (-323.706, -93.9378, 10) construction
  line L192 (-263.7718, -62.3378, 10) -> (-263.7718, -49.3378, 10)
  arc A211 through (-27.2405, -67.8878, 10) (-27.5941, -68.0342, 10) (-27.7405, -68.3878, 10)
  arc A212 through (-14.2405, -81.8878, 10) (-13.8869, -81.7413, 10) (-13.7405, -81.3878, 10)
  line L193 (-276.178, -10.7378, 10) -> (-289.178, -10.7378, 10)
  line L194 (-176.1655, -48.8378, 10) -> (-189.1655, -48.8378, 10)
  line L195 (-195.2155, -62.8378, 10) -> (-208.2155, -62.8378, 10)
  line L196 (-233.3155, -62.8378, 10) -> (-246.3155, -62.8378, 10)
  line L197 (-204.7405, -29.7878, 10) -> (-217.7405, -29.7878, 10)
  line L198 (-270.628, -24.2378, 10) -> (-270.628, -11.2378, 10)
  arc A213 through (-279.653, -86.9378, 10) (-280.0066, -87.0842, 10) (-280.153, -87.4378, 10)
  arc A214 through (-61.078, -100.4378, 10) (-60.9316, -100.7913, 10) (-60.578, -100.9378, 10)
  line L199 (-84.4218, -23.7378, 10) -> (-90.4218, -23.7378, 10)
  line L200 (-199.978, -10.7378, 10) -> (-212.978, -10.7378, 10)
  arc A215 through (-199.978, -100.9378, 10) (-199.6244, -100.7913, 10) (-199.478, -100.4378, 10)
  arc A216 through (-28.028, -87.4378, 10) (-28.1744, -87.0842, 10) (-28.528, -86.9378, 10)
  arc A217 through (-180.428, -87.4378, 10) (-180.5744, -87.0842, 10) (-180.928, -86.9378, 10)
  arc A218 through (-176.1655, -124.7503, 10) (-175.8119, -124.6038, 10) (-175.6655, -124.2503, 10)
  line L201 (-295.228, -43.7878, 10) -> (-308.228, -43.7878, 10)
  line L202 (-185.6905, -29.7878, 10) -> (-198.6905, -29.7878, 10)
  line L203 (-199.1905, -43.2878, 10) -> (-199.1905, -30.2878, 10)
  line L204 (-219.028, -10.7378, 10) -> (-232.028, -10.7378, 10)
  arc A219 through (-156.6155, -111.2503, 10) (-156.7619, -110.8967, 10) (-157.1155, -110.7503, 10)
  line L205 (-83.9218, -23.2378, 10) -> (-83.9218, -9.2378, 10)
  line L206 (-158.853, -141.488, 10) -> (-158.853, -132.2753, 10) construction
  arc A220 through (-127.253, -110.7503, 10) (-127.6066, -110.8967, 10) (-127.753, -111.2503, 10)
  line L207 (-15.978, -124.7503, 10) -> (-15.978, -141.488, 10) construction
  arc A221 through (-195.2155, -124.7503, 10) (-194.8619, -124.6038, 10) (-194.7155, -124.2503, 10)
  arc A222 through (-161.878, -100.9378, 10) (-161.5244, -100.7913, 10) (-161.378, -100.4378, 10)
  arc A223 through (-189.1655, -110.7503, 10) (-189.5191, -110.8967, 10) (-189.6655, -111.2503, 10)
  line L208 (-213.478, -24.2378, 10) -> (-213.478, -11.2378, 10)
  arc A224 through (-136.778, -86.9378, 10) (-137.1316, -87.0842, 10) (-137.278, -87.4378, 10)
  arc A225 through (-9.478, -124.7503, 10) (-9.1244, -124.6038, 10) (-8.978, -124.2503, 10)
  arc A226 through (-155.828, -86.9378, 10) (-156.1816, -87.0842, 10) (-156.328, -87.4378, 10)
  line L209 (-294.728, -43.2878, 10) -> (-294.728, -30.2878, 10)
  line L210 (-49.1718, -24.2378, 10) -> (-49.1718, -11.2378, 10)
  arc A227 through (-8.978, -111.2503, 10) (-9.1244, -110.8967, 10) (-9.478, -110.7503, 10)
  arc A228 through (-114.253, -124.7503, 10) (-113.8994, -124.6038, 10) (-113.753, -124.2503, 10)
  arc A229 through (-170.1155, -110.7503, 10) (-170.4691, -110.8967, 10) (-170.6155, -111.2503, 10)
  arc A230 through (-118.228, -100.4378, 10) (-118.0816, -100.7913, 10) (-117.728, -100.9378, 10)
  arc A231 through (-219.028, -124.7503, 10) (-218.6744, -124.6038, 10) (-218.528, -124.2503, 10)
  line L211 (-237.2905, -43.2878, 10) -> (-237.2905, -30.2878, 10)
  arc A232 through (-270.628, -124.2503, 10) (-270.4816, -124.6038, 10) (-270.128, -124.7503, 10)
  arc A233 through (-85.178, -87.4378, 10) (-85.3244, -87.0842, 10) (-85.678, -86.9378, 10)
  arc A234 through (-66.128, -87.4378, 10) (-66.2744, -87.0842, 10) (-66.628, -86.9378, 10)
  arc A235 through (-232.028, -110.7503, 10) (-232.3816, -110.8967, 10) (-232.528, -111.2503, 10)
  line L212 (-237.578, -24.2378, 10) -> (-237.578, -11.2378, 10)
  line L213 (-118.5155, -62.3378, 10) -> (-118.5155, -49.3378, 10)
  line L214 (-180.428, -100.4378, 10) -> (-180.428, -87.4378, 10)
  line L215 (-127.753, -81.3878, 10) -> (-127.753, -68.3878, 10)
  line L216 (-264.715, -99.4378, 10) -> (-264.715, -85.4378, 10)
  arc A236 through (-35.6718, -24.7378, 10) (-35.3182, -24.5913, 10) (-35.1718, -24.2378, 10)
  arc A237 through (-137.5655, -49.3378, 10) (-137.7119, -48.9842, 10) (-138.0655, -48.8378, 10)
  arc A238 through (-251.578, -24.2378, 10) (-251.4316, -24.5913, 10) (-251.078, -24.7378, 10)
  line L217 (-114.253, -81.8878, 10) -> (-127.253, -81.8878, 10)
  line L218 (6, -67.744, 10) -> (-6.453, -67.744, 10) construction
  line L219 (-184.4218, -8.7378, 10) -> (-190.4218, -8.7378, 10)
  arc A239 through (-289.178, -10.7378, 10) (-289.5316, -10.8842, 10) (-289.678, -11.2378, 10)
  line L220 (-21.3843, -43.7878, 10) -> (-34.3843, -43.7878, 10)
  line L221 (-249.4843, -43.2878, 10) -> (-249.4843, -30.2878, 10)
  arc A240 through (-213.478, -24.2378, 10) (-213.3316, -24.5913, 10) (-212.978, -24.7378, 10)
  arc A241 through (-277.7718, -62.3378, 10) (-277.6253, -62.6913, 10) (-277.2718, -62.8378, 10)
  line L222 (-65.8405, -43.2878, 10) -> (-65.8405, -30.2878, 10)
  arc A242 through (-156.6155, -49.3378, 10) (-156.7619, -48.9842, 10) (-157.1155, -48.8378, 10)
  arc A243 through (-24.8593, -10.7378, 10) (-25.2128, -10.8842, 10) (-25.3593, -11.2378, 10)
  arc A244 through (-275.678, -11.2378, 10) (-275.8244, -10.8842, 10) (-276.178, -10.7378, 10)
  line L223 (-132.803, -81.3878, 10) -> (-132.803, -68.3878, 10)
  arc A245 through (-233.3155, -62.8378, 10) (-232.9619, -62.6913, 10) (-232.8155, -62.3378, 10)
  line L224 (-295.228, -24.7378, 10) -> (-308.228, -24.7378, 10)
  line L225 (-12.4463, -42.2878, 10) -> (-12.4463, -28.2878, 10)
  line L226 (-132.5155, -62.3378, 10) -> (-132.5155, -49.3378, 10)
  arc A246 through (-237.578, -11.2378, 10) (-237.7244, -10.8842, 10) (-238.078, -10.7378, 10)
  line L227 (-94.703, -81.3878, 10) -> (-94.703, -68.3878, 10)
  line L228 (-76.153, -81.8878, 10) -> (-89.153, -81.8878, 10)
  line L229 (-199.978, -86.9378, 10) -> (-212.978, -86.9378, 10)
  arc A247 through (-179.6405, -29.7878, 10) (-179.9941, -29.9342, 10) (-180.1405, -30.2878, 10)
  line L230 (-279.7098, -46.8378, 10) -> (-285.7098, -46.8378, 10)
  arc A248 through (-119.0155, -62.8378, 10) (-118.6619, -62.6913, 10) (-118.5155, -62.3378, 10)
  line L231 (-213.478, -100.4378, 10) -> (-213.478, -87.4378, 10)
  line L232 (-223.7905, -43.7878, 10) -> (-236.7905, -43.7878, 10)
  arc A249 through (-144.4218, -24.2378, 10) (-144.2753, -24.5913, 10) (-143.9218, -24.7378, 10)
  line L233 (-247.603, -67.8878, 10) -> (-260.603, -67.8878, 10)
  line L234 (-223.003, -81.3878, 10) -> (-223.003, -68.3878, 10)
  line L235 (-219.028, -100.9378, 10) -> (-232.028, -100.9378, 10)
  line L236 (-271.4155, -81.8878, 10) -> (-284.4155, -81.8878, 10)
  line L237 (-144.4218, -24.2378, 10) -> (-144.4218, -11.2378, 10)
  line L238 (-151.853, -81.3878, 10) -> (-151.853, -68.3878, 10)
  line L239 (-203.953, -81.3878, 10) -> (-203.953, -68.3878, 10)
  arc A250 through (-241.553, -67.8878, 10) (-241.9066, -68.0342, 10) (-242.053, -68.3878, 10)
  arc A251 through (-166.1405, -30.2878, 10) (-166.2869, -29.9342, 10) (-166.6405, -29.7878, 10)
  line L240 (-255.3338, -61.3378, 10) -> (-255.3338, -47.3378, 10)
  arc A252 through (-89.9405, -30.2878, 10) (-90.0869, -29.9342, 10) (-90.4405, -29.7878, 10)
  line L241 (-130.9218, -10.7378, 10) -> (-143.9218, -10.7378, 10)
  arc A253 through (-184.403, -67.8878, 10) (-184.7566, -68.0342, 10) (-184.903, -68.3878, 10)
  line L242 (-204.7405, -43.7878, 10) -> (-217.7405, -43.7878, 10)
  arc A254 through (-184.903, -81.3878, 10) (-184.7566, -81.7413, 10) (-184.403, -81.8878, 10)
  line L243 (-284.9155, -81.3878, 10) -> (-284.9155, -68.3878, 10)
  line L244 (-147.0905, -43.2878, 10) -> (-147.0905, -30.2878, 10)
  line L245 (-219.028, -86.9378, 10) -> (-232.028, -86.9378, 10)
  arc A255 through (-49.1718, -24.2378, 10) (-49.0253, -24.5913, 10) (-48.6718, -24.7378, 10)
  arc A256 through (-152.353, -81.8878, 10) (-151.9994, -81.7413, 10) (-151.853, -81.3878, 10)
  line L246 (-166.6405, -43.7878, 10) -> (-179.6405, -43.7878, 10)
  line L247 (-130.9218, -24.7378, 10) -> (-143.9218, -24.7378, 10)
  line L248 (-133.303, -67.8878, 10) -> (-146.303, -67.8878, 10)
  line L249 (-294.728, -81.3878, 10) -> (-294.728, -68.3878, 10)
  arc A257 through (-72.9843, -24.2378, 10) (-72.8378, -24.5913, 10) (-72.4843, -24.7378, 10)
  arc A258 through (-199.978, -24.7378, 10) (-199.6244, -24.5913, 10) (-199.478, -24.2378, 10)
  line L250 (-61.8655, -62.8378, 10) -> (-74.8655, -62.8378, 10)
  line L251 (-166.1405, -43.2878, 10) -> (-166.1405, -30.2878, 10)
  line L252 (-57.103, -81.8878, 10) -> (-70.103, -81.8878, 10)
  arc A259 through (-35.1718, -11.2378, 10) (-35.3182, -10.8842, 10) (-35.6718, -10.7378, 10)
  arc A260 through (-84.8905, -43.2878, 10) (-84.7441, -43.6413, 10) (-84.3905, -43.7878, 10)
  arc A261 through (-51.8405, -30.2878, 10) (-51.9869, -29.9342, 10) (-52.3405, -29.7878, 10)
  line L253 (-238.078, -86.9378, 10) -> (-251.078, -86.9378, 10)
  arc A262 through (-52.3405, -43.7878, 10) (-51.9869, -43.6413, 10) (-51.8405, -43.2878, 10)
  line L254 (-75.3655, -62.3378, 10) -> (-75.3655, -49.3378, 10)
  arc A263 through (-294.728, -30.2878, 10) (-294.8744, -29.9342, 10) (-295.228, -29.7878, 10)
  line L255 (-247.103, -81.3878, 10) -> (-247.103, -68.3878, 10)
  arc A264 through (-236.7905, -29.7878, 10) (-237.1441, -29.9342, 10) (-237.2905, -30.2878, 10)
  line L256 (-137.5655, -62.3378, 10) -> (-137.5655, -49.3378, 10)
  arc A265 through (-160.5905, -29.7878, 10) (-160.9441, -29.9342, 10) (-161.0905, -30.2878, 10)
  line L257 (-189.953, -81.3878, 10) -> (-189.953, -68.3878, 10)
  arc A266 through (-279.2098, -47.3378, 10) (-279.3562, -46.9842, 10) (-279.7098, -46.8378, 10)
  line L258 (-34.8843, -43.2878, 10) -> (-34.8843, -30.2878, 10)
  arc A267 through (-261.8338, -46.8378, 10) (-262.1873, -46.9842, 10) (-262.3338, -47.3378, 10)
  arc A268 through (-123.778, -100.9378, 10) (-123.4244, -100.7913, 10) (-123.278, -100.4378, 10)
  line L259 (-152.353, -81.8878, 10) -> (-165.353, -81.8878, 10)
  arc A269 through (-180.928, -100.9378, 10) (-180.5744, -100.7913, 10) (-180.428, -100.4378, 10)
  arc A270 through (-128.0405, -30.2878, 10) (-128.1869, -29.9342, 10) (-128.5405, -29.7878, 10)
  line L260 (-11.8593, -24.7378, 10) -> (-24.8593, -24.7378, 10)
  line L261 (-113.4655, -62.3378, 10) -> (-113.4655, -49.3378, 10)
  arc A271 through (-103.4405, -29.7878, 10) (-103.7941, -29.9342, 10) (-103.9405, -30.2878, 10)
  line L262 (-19.4463, -42.2878, 10) -> (-19.4463, -28.2878, 10)
  arc A272 through (-109.4905, -43.7878, 10) (-109.1369, -43.6413, 10) (-108.9905, -43.2878, 10)
  arc A273 through (-262.3338, -61.3378, 10) (-262.1873, -61.6913, 10) (-261.8338, -61.8378, 10)
  line L263 (-119.0155, -62.8378, 10) -> (-132.0155, -62.8378, 10)
  line L264 (-12.9463, -27.7878, 10) -> (-18.9463, -27.7878, 10)
  arc A274 through (-42.8223, -27.7878, 10) (-43.1758, -27.9342, 10) (-43.3223, -28.2878, 10)
  line L265 (-16.6218, -62.8378, 10) -> (-29.6218, -62.8378, 10)
  line L266 (-85.678, -100.9378, 10) -> (-98.678, -100.9378, 10)
  line L267 (-35.1718, -24.2378, 10) -> (-35.1718, -11.2378, 10)
  line L268 (-170.903, -81.3878, 10) -> (-170.903, -68.3878, 10)
  arc A275 through (-66.628, -100.9378, 10) (-66.2744, -100.7913, 10) (-66.128, -100.4378, 10)
  line L269 (-25.3593, -24.2378, 10) -> (-25.3593, -11.2378, 10)
  arc A276 through (-47.578, -100.9378, 10) (-47.2244, -100.7913, 10) (-47.078, -100.4378, 10)
  line L270 (-209.503, -81.8878, 10) -> (-222.503, -81.8878, 10)
  arc A277 through (-189.6655, -124.2503, 10) (-189.5191, -124.6038, 10) (-189.1655, -124.7503, 10)
  arc A278 through (-289.178, -110.7503, 10) (-289.5316, -110.8967, 10) (-289.678, -111.2503, 10)
  arc A279 through (-156.328, -100.4378, 10) (-156.1816, -100.7913, 10) (-155.828, -100.9378, 10)
  arc A280 through (-251.078, -110.7503, 10) (-251.4316, -110.8967, 10) (-251.578, -111.2503, 10)
  line L271 (-271.4155, -67.8878, 10) -> (-284.4155, -67.8878, 10)
  arc A281 through (-275.678, -111.2503, 10) (-275.8244, -110.8967, 10) (-276.178, -110.7503, 10)
  line L272 (-266.653, -86.9378, 10) -> (-279.653, -86.9378, 10)
  line L273 (-258.215, -99.9378, 10) -> (-264.215, -99.9378, 10)
  line L274 (-75.653, -81.3878, 10) -> (-75.653, -68.3878, 10)
  line L275 (-308.728, -24.2378, 10) -> (-308.728, -11.2378, 10)
  circle A282 through (-0.5, 2.5, 10) (4, -0.0981, 10) (4, 5.0981, 10)
  line L276 (-232.528, -24.2378, 10) -> (-232.528, -11.2378, 10)
  line L277 (-138.0655, -62.8378, 10) -> (-151.0655, -62.8378, 10)
  line L278 (-166.6405, -29.7878, 10) -> (-179.6405, -29.7878, 10)
  line L279 (-280.153, -100.4378, 10) -> (-280.153, -87.4378, 10)
  line L280 (-294.728, -100.4378, 10) -> (-294.728, -87.4378, 10)
  line L281 (-8.978, -117.7503, 10) -> (6, -117.7503, 10) construction
  arc A283 through (-289.678, -124.2503, 10) (-289.5316, -124.6038, 10) (-289.178, -124.7503, 10)
  line L282 (-185.6905, -43.7878, 10) -> (-198.6905, -43.7878, 10)
  arc A284 through (-208.7155, -124.2503, 10) (-208.5691, -124.6038, 10) (-208.2155, -124.7503, 10)
  line L283 (-61.8655, -48.8378, 10) -> (-74.8655, -48.8378, 10)
  line L284 (-137.278, -100.4378, 10) -> (-137.278, -87.4378, 10)
  arc A285 through (-151.0655, -110.7503, 10) (-151.4191, -110.8967, 10) (-151.5655, -111.2503, 10)